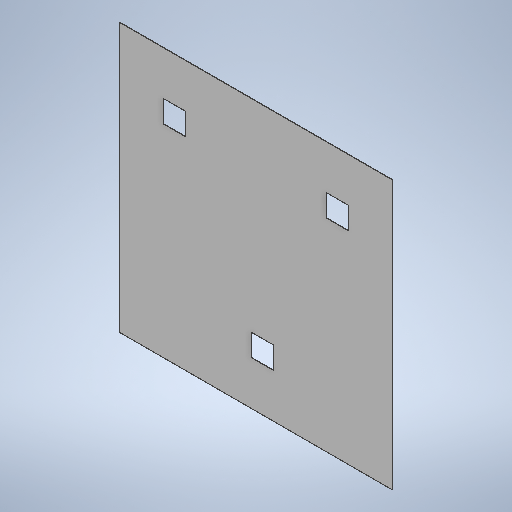
# Autodesk Inventor part: Heat sheild
Saved by Autodesk Inventor 2025.1 (Build 291241020, 241B)
## iProperties
Created: 2024-09-24
Part Number: Heat sheild
Material: Generic
Document SubType Name: Modeling
Designer: jjk
Density: 1 g/cm^3
Appearance: Default
Author: jjk
Autodesk Inventor part; units mm, degrees
ref_plane "YZ Plane" through (0, 0, 0) normal (1, 0, 0) x (0, 1, 0)
ref_plane "XZ Plane" through (0, 0, 0) normal (0, 1, 0) x (-1, 0, 0)
ref_plane "XY Plane" through (0, 0, 0) normal (0, 0, 1) x (1, 0, 0)
sketch "Sketch1" plane through (0, 0, 0) normal (0, 0, 1) x (1, 0, 0)
  line L0 (0, 0) -> (157.48, 0)
  line L1 (157.48, 0) -> (157.48, 154.94)
  line L2 (0, 154.94) -> (0, 0)
  line L3 (61.8236, 154.94) -> (18.6436, 154.94)
  line L4 (11.0236, 154.94) -> (0, 154.94)
  line L5 (157.48, 154.94) -> (120.2436, 154.94)
  line L6 (112.6236, 154.94) -> (69.4436, 154.94)
  line L7 (11.0236, 154.94) -> (18.6436, 154.94)
  line L8 (61.8236, 154.94) -> (69.4436, 154.94)
  line L9 (120.2436, 154.94) -> (112.6236, 154.94)
  line L10 (25.4, 129.54) -> (38.1, 129.54)
  line L11 (38.1, 129.54) -> (38.1, 116.84)
  line L12 (38.1, 116.84) -> (25.4, 116.84)
  line L13 (25.4, 116.84) -> (25.4, 129.54)
  line L14 (119.38, 129.54) -> (132.08, 129.54)
  line L15 (132.08, 129.54) -> (132.08, 116.84)
  line L16 (132.08, 116.84) -> (119.38, 116.84)
  line L17 (119.38, 116.84) -> (119.38, 129.54)
  line L18 (76.2, 38.1) -> (88.9, 38.1)
  line L19 (88.9, 38.1) -> (88.9, 25.4)
  line L20 (88.9, 25.4) -> (76.2, 25.4)
  line L21 (76.2, 25.4) -> (76.2, 38.1)
  dimension "d0" = 154.94
  dimension "d1" = 157.48
  dimension "d19" = 12.7
  dimension "d20" = 12.7
  dimension "d21" = 12.7
  dimension "d22" = 12.7
  dimension "d23" = 12.7
  dimension "d24" = 25.4
  dimension "d25" = 25.4
  dimension "d26" = 76.2
  dimension "d27" = 25.4
  dimension "d28" = 25.4
  constraints: 44 end point, 11 parallel, 5 horizontal, 4 perpendicular, 2 collinear, 2 point on line
  measures "d0" distance of L0.end L1.end
  measures "d1" distance of L0.start L0.end
  measures "d19" distance of L12.end L10.start
  measures "d20" distance of L10.start L10.end
  measures "d21" distance of L14.start L14.end
  measures "d22" distance of L18.start L18.end
  measures "d23" distance of L20.end L18.start
  measures "d24" distance between parallel lines of L2 L13
  measures "d25" distance between parallel lines of L1 L15
  measures "d26" distance between parallel lines of L2 L21
  measures "d27" distance between parallel lines of L0 L20
  measures "d28" distance between parallel lines of L3 L10
extrude "Extrusion1" add sketch "Sketch1" along normal blind 0.254
body "Solid1"
